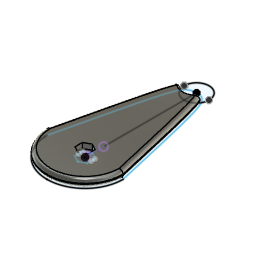
DiscoCame_newVersion_novoProjeto (Autodesk Fusion 360 design; units mm, degrees)
Autodesk Fusion 360 part; units mm, degrees
sketch "Esboço1" plane through (0, 0, 0) normal (0, 0, 1) x (1, 0, 0)
  circle A0 centre (0, 0) radius 2
  arc A1 (0, -46) -> (46, 0) centre (0, 0) ccw
  arc A2 (-46, 0) -> (0, -46) centre (0, 0) ccw
  line L0 (0, 0) -> (0, 135)
  spline S0 degree 2 poles (-46, 0) (-15, 135) (0, 135) knots 0 0 0 14.558611 14.558611 14.558611 weights 1 3 1
  spline S1 degree 2 poles (46, 0) (15, 135) (0, 135) knots 0 0 0 14.558611 14.558611 14.558611 weights 1 3 1
  circle A3 centre (0, 135) radius 15
  line L1 (0, 1.75) -> (0, 22.5)
  line L2 (7.65, 0) -> (7.65, 4.4165)
  line L3 (7.65, 0) -> (7.65, 4.4165)
  line L4 (7.65, 0) -> (7.65, -4.4165)
  line L5 (-7.65, 0) -> (-7.65, 4.4165)
  line L6 (-7.65, 0) -> (-7.65, 4.4165)
  line L7 (-7.65, 0) -> (-7.65, -4.4165)
  line L8 (-7.65, 4.4165) -> (0, 8.833)
  line L9 (0, 8.833) -> (7.65, 4.4165)
  line L10 (-7.65, -4.4165) -> (0, -8.833)
  line L11 (0, -8.833) -> (7.65, -4.4165)
  dimension "d1" = 4
  dimension "d9" = 46
  dimension "d34" = 30
  dimension "d35" = 135
  constraint coincident A0.centre A1.centre
  constraint vertical L0
  constraint coincident L0.end L1
  constraint coincident L0.end S0.end
  measures "d1" diameter of A0
  measures "d9" radius of A1
  measures "d34" diameter of A3
  measures "d35" distance of A0.centre L0.end
extrude "Extrusão3" add sketch "Esboço1" along normal blind 9.5 contours A1 A2 S0 S1 A3
extrude "Extrusão4" add sketch "Esboço1" along normal blind 3 contours L2 L3 L4 L5 L6 L7 L8 L9 L10 L11
fillet "Arredondamento9" radius 4.25 6 edges at (21.2239, 103.9308, 9.5) (21.2239, 103.9308, 0) (0, -46, 9.5) (0, -46, 0) (-21.2239, 103.9308, 9.5) (-21.2239, 103.9308, 0)
fillet "Arredondamento10" radius 2 8 edges at (-13.0208, 127.5529, 4.75) (-12.2362, 126.324, 1.2102) (0, 120, 0) (12.2346, 126.3217, 1.2078) (13.0208, 127.5529, 4.75) (12.2362, 126.324, 8.2898) (0, 120, 9.5) (-12.2346, 126.3217, 8.2922)
equation "d35 = 150 mm - d34 / 2"
